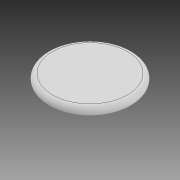
# Autodesk Inventor part: RegulatorValve
Saved by Autodesk Inventor 2020 (Build 240168000, 168)
## iProperties
Created: 2021-05-21
Part Number: RegulatorValve
Material: Generic
Document SubType Name: Modeling
Designer: DDeGo
Density: 1 g/cm^3
Appearance: Default
Author: DDeGo
Autodesk Inventor part; units mm, degrees
ref_plane "YZ Plane" through (0, 0, 0) normal (1, 0, 0) x (0, 1, 0)
ref_plane "XZ Plane" through (0, 0, 0) normal (0, 1, 0) x (-1, 0, 0)
ref_plane "XY Plane" through (0, 0, 0) normal (0, 0, 1) x (1, 0, 0)
sketch "Sketch1" plane through (0, 0, 0) normal (0, 0, 1) x (1, 0, 0)
  line L0 (0, 0) -> (0, 4.7)
  line L1 (0, 4.7) -> (6.25, 4.7)
  line L2 (6.25, 3.2) -> (2.5, 3.2)
  line L3 (2.5, 3.2) -> (1.5, 2.836)
  line L4 (1.5, 2.836) -> (1.5, 0.3541)
  arc A0 (6.25, 3.2) -> (6.25, 4.7) centre (6.25, 3.95) ccw
  arc A1 (0.8571, -0.1251) -> (1.5, 0.3541) centre (1, 0.3541) ccw
  arc A2 (0.8571, -0.1251) -> (0, 0) centre (0, -3) ccw
  dimension "d0" = 1.5
  dimension "d4" = 1.5
  dimension "d9" = 7
  dimension "d13" = 0.5
  dimension "d15" = 2.5
  dimension "d16" = 3
  dimension "d17" = 3.2
  dimension "d33" = 160
  constraints: 14 end point, 6 point on circle, 4 tangent, 3 centre point, 1 parallel, 1 perpendicular, 1 point on line, 1 vertical
  measures "d0" distance between parallel lines of L0 L4
  measures "d4" distance between parallel lines of L1 L2
  measures "d13" radius of A1
  measures "d15" distance from line of L0 L2.end
  measures "d16" radius of A2
  measures "d17" distance from line of L0.start L2
  measures "d33" angle of L2 L3
revolve "Revolution1" add sketch "Sketch1" angle 360 about axis through (0, 0, 0) along (0, 1, 0)
sketch "Sketch2" plane through (0, 0, 0) normal (0, 1, 0) x (-1, 0, 0)
  circle A0 centre (0, 0) radius 1.5 construction
  line L0 (0, -1.4) -> (0, -1.6) construction
  line L1 (-0.4, -1.4) -> (-0.4, -1.6)
  line L2 (0.4, -1.6) -> (0.4, -1.4)
  arc A1 (0.4, -1.4) -> (-0.4, -1.4) centre (0, -1.4) ccw
  arc A2 (-0.4, -1.6) -> (0.4, -1.6) centre (0, -1.6) ccw
  line L3 (1.3315, -0.4326) -> (1.5217, -0.4944) construction
  line L4 (1.2079, -0.813) -> (1.3981, -0.8748)
  line L5 (1.6453, -0.114) -> (1.4551, -0.0522)
  arc A3 (1.4551, -0.0522) -> (1.2079, -0.813) centre (1.3315, -0.4326) ccw
  arc A4 (1.3981, -0.8748) -> (1.6453, -0.114) centre (1.5217, -0.4944) ccw
  line L6 (0.8229, 1.1326) -> (0.9405, 1.2944) construction
  line L7 (1.1465, 0.8975) -> (1.2641, 1.0593)
  line L8 (0.6168, 1.5295) -> (0.4993, 1.3677)
  arc A5 (0.4993, 1.3677) -> (1.1465, 0.8975) centre (0.8229, 1.1326) ccw
  arc A6 (1.2641, 1.0593) -> (0.6168, 1.5295) centre (0.9405, 1.2944) ccw
  line L9 (-0.8229, 1.1326) -> (-0.9405, 1.2944) construction
  line L10 (-0.4993, 1.3677) -> (-0.6168, 1.5295)
  line L11 (-1.2641, 1.0593) -> (-1.1465, 0.8975)
  arc A7 (-1.1465, 0.8975) -> (-0.4993, 1.3677) centre (-0.8229, 1.1326) ccw
  arc A8 (-0.6168, 1.5295) -> (-1.2641, 1.0593) centre (-0.9405, 1.2944) ccw
  line L12 (-1.3315, -0.4326) -> (-1.5217, -0.4944) construction
  line L13 (-1.4551, -0.0522) -> (-1.6453, -0.114)
  line L14 (-1.3981, -0.8748) -> (-1.2079, -0.813)
  arc A9 (-1.2079, -0.813) -> (-1.4551, -0.0522) centre (-1.3315, -0.4326) ccw
  arc A10 (-1.6453, -0.114) -> (-1.3981, -0.8748) centre (-1.5217, -0.4944) ccw
  point P0 (0, 0)
  point P1 (0, -1.5)
  point P2 (0, 0)
  point P3 (1.4266, -0.4635)
  point P4 (0, 0)
  point P5 (0.8817, 1.2135)
  point P6 (0, 0)
  point P7 (-0.8817, 1.2135)
  point P8 (0, 0)
  point P9 (-1.4266, -0.4635)
  dimension "d23" = 0.8
  dimension "d24" = 0.2
  dimension "d27" = 360
  constraints: 40 end point, 20 point on circle, 10 centre point, 5 point on line, 4 tangent, 2 coincident, 1 midpoint, 1 parallel, 1 vertical, 1 vertical alignment, 65 other
  measures "d23" distance between parallel lines of L2 L1
  measures "d24" distance of L0.start L0.end
extrude "Extrusion1" cut sketch "Sketch2" along normal up to surface round surface about axis through (0, 3.018, 0) along (0, -1, 0) radius 2 half angle -70 far side no
extrude "Extrusion2" cut sketch "Sketch2" against normal blind 10
body "Solid1"
